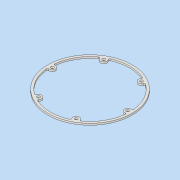
# Autodesk Inventor part: PreloadSpacerForThreadedRods
Saved by Autodesk Inventor 2017 (Build 210142000, 142)
## iProperties
Created: 2019-07-18
Part Number: PreloadSpacerForThreadedRods
Material: ABS Plastic
Document SubType Name: Modeling
Designer: techn
Density: 1.06 g/cm^3
Appearance: Smooth - White
Author: techn
Autodesk Inventor part; units mm, degrees
ref_plane "YZ Plane" through (0, 0, 0) normal (1, 0, 0) x (0, 1, 0)
ref_plane "XZ Plane" through (0, 0, 0) normal (0, 1, 0) x (-1, 0, 0)
ref_plane "XY Plane" through (0, 0, 0) normal (0, 0, 1) x (1, 0, 0)
sketch "Sketch1" plane through (0, 0, 0) normal (0, 1, 0) x (-1, 0, 0)
  circle A0 centre (0, 0) radius 46.736
  circle A1 centre (0, 0) radius 44.196
  circle A2 centre (41.91, 0) radius 1.651
  circle A3 centre (41.91, 0) radius 3.4925
  circle A4 centre (20.955, 36.2951) radius 1.651
  circle A5 centre (20.955, 36.2951) radius 3.4925
  circle A6 centre (-20.955, 36.2951) radius 1.651
  circle A7 centre (-20.955, 36.2951) radius 3.4925
  circle A8 centre (-41.91, 0) radius 1.651
  circle A9 centre (-41.91, 0) radius 3.4925
  circle A10 centre (-20.955, -36.2951) radius 1.651
  circle A11 centre (-20.955, -36.2951) radius 3.4925
  circle A12 centre (20.955, -36.2951) radius 1.651
  circle A13 centre (20.955, -36.2951) radius 3.4925
  dimension "d0" = 93.472
  dimension "d1" = 88.392
  dimension "d2" = 3.302
  dimension "d3" = 6.985
  dimension "d4" = 41.91
  dimension "d7" = 360
  constraints: 14 centre point, 8 coincident, 25 other
  measures "d0" diameter of A0
  measures "d1" diameter of A1
  measures "d2" diameter of A2
  measures "d3" diameter of A3
  measures "d4" distance of point (0, 0) A2.centre
extrude "Extrusion1" add sketch "Sketch1" along normal blind 1.905 contours A0 | A1 A3 | A1 A3 | A5 A1 | A1 A5 | A13 A1 | A1 A13 | A7 A1 | A1 A7 | A11 A1 | A1 A11 | A9 A1 | A1 A9
fillet "Fillet1" radius 1.27 2 edges at (-44.1128, 0.9525, 2.7102) (-44.1128, 0.9525, -2.7102)
pattern_circular "Circular Pattern1" count 6 over 360 about axis through (0, 0, 0) along (0, 1, 0) of "Fillet1"
body "Solid1"
